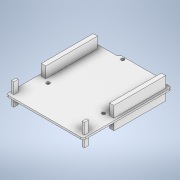
# Autodesk Inventor part: Microcontroller
Saved by Autodesk Inventor 2022 (Build 260153000, 153)
## iProperties
Created: 2022-02-18
Part Number: Microcontroller
Material: Generic
Document SubType Name: Modeling
Designer: woutr
Density: 1 g/cm^3
Appearance: White
Author: woutr
Autodesk Inventor part; units mm, degrees
ref_plane "YZ Plane" through (0, 0, 0) normal (1, 0, 0) x (0, 1, 0)
ref_plane "XZ Plane" through (0, 0, 0) normal (0, 1, 0) x (-1, 0, 0)
ref_plane "XY Plane" through (0, 0, 0) normal (0, 0, 1) x (1, 0, 0)
sketch "Sketch1" plane through (0, 0, 0) normal (0, 1, 0) x (-1, 0, 0)
  line L0 (0, 0) -> (70, 0)
  line L1 (70, 0) -> (70, -80.5)
  line L2 (70, -80.5) -> (49.49, -80.5)
  line L3 (0, 0) -> (0, -80.5)
  line L4 (0, -80.5) -> (11.33, -80.5)
  line L5 (47.54, -82.45) -> (13.28, -82.45)
  line L6 (49.49, -80.5) -> (47.54, -82.45)
  line L7 (11.33, -80.5) -> (13.28, -82.45)
  dimension "d0" = 70
  dimension "d1" = 80.5
  dimension "d2" = 20.51
  dimension "d3" = 80.5
  dimension "d4" = 11.33
  dimension "d5" = 82.45
  dimension "d6" = 45
  dimension "d7" = 45
  constraints: 16 end point, 3 perpendicular, 2 horizontal, 1 vertical
  measures "d0" distance of L0.start L0.end
  measures "d1" distance of L0.end L1.end
  measures "d2" distance of L1.end L2.end
  measures "d3" distance of L0.start L3.end
  measures "d4" distance of L3.end L4.end
  measures "d5" distance between parallel lines of L0 L5
  measures "d6" angle of L2 L6
  measures "d7" angle of L4 L7
extrude "Extrusion1" add sketch "Sketch1" along normal blind 1.65
fillet "Fillet1" radius 2 4 edges at (0, 0.825, 0) (-70, 0.825, 0) (0, 0.825, -80.5) (-70, 0.825, -80.5)
sketch "Sketch2" plane through (0, 1.65, 0) normal (0, 1, 0) x (1, 0, 0)
  circle A0 centre (-59.5, 27.7) radius 1.5
  circle A1 centre (-10.5, 29) radius 1.5
  circle A2 centre (-44.2, 80.15) radius 1.5
  line L0 (-68, 0) -> (-2, 0) projected
  line L1 (0, 2) -> (0, 78.5) projected
  line L2 (-70, 78.5) -> (-70, 2) projected
  line L3 (-13.28, 82.45) -> (-47.54, 82.45) projected
  point P0 (0, 0)
  dimension "d11" = 3
  dimension "d12" = 3
  dimension "d13" = 3
  dimension "d14" = 29
  dimension "d15" = 10.5
  dimension "d16" = 10.5
  dimension "d17" = 2.3
  dimension "d18" = 25.8
  dimension "d40" = 27.7
  constraints: 3 centre point
  measures "d11" diameter of A0
  measures "d12" diameter of A1
  measures "d13" diameter of A2
  measures "d14" distance from line of L0 A1.centre
  measures "d15" distance from line of L1 A1.centre
  measures "d16" distance from line of L2 A0.centre
  measures "d17" distance from line of L3 A2.centre
  measures "d18" distance from line of L2 A2.centre
  measures "d40" distance from line of L0 A0.centre
extrude "Extrusion2" cut sketch "Sketch2" against normal through all
sketch "Sketch3" plane through (0, 0, 0) normal (0, -1, 0) x (1, 0, 0)
  line L0 (-2, -30) -> (-6, -30)
  line L1 (-6, -30) -> (-6, -77)
  line L2 (-6, -77) -> (-2, -77)
  line L3 (-2, -77) -> (-2, -30)
  line L4 (-68, 0) -> (-2, 0) projected
  line L5 (0, -2) -> (0, -78.5) projected
  line L6 (-64, -30) -> (-68, -30)
  line L7 (-68, -30) -> (-68, -77)
  line L8 (-68, -77) -> (-64, -77)
  line L9 (-64, -77) -> (-64, -30)
  line L10 (-70, -78.5) -> (-70, -2) projected
  line L11 (-49.49, -80.5) -> (-68, -80.5) projected
  line L12 (-2, -7) -> (-4, -7)
  line L13 (-4, -7) -> (-4, -3)
  line L14 (-4, -3) -> (-2, -3)
  line L15 (-2, -3) -> (-2, -7)
  line L16 (-66, -7) -> (-68, -7)
  line L17 (-68, -7) -> (-68, -3)
  line L18 (-68, -3) -> (-66, -3)
  line L19 (-66, -3) -> (-66, -7)
  point P0 (0, 0)
  point P1 (-4, -77)
  point P2 (-66, -77)
  point P3 (-2, -5)
  point P4 (-68, -5)
  point P5 (-3, -3)
  point P6 (-67, -3)
  dimension "d21" = 4
  dimension "d22" = 47
  dimension "d23" = 30
  dimension "d24" = 2
  dimension "d27" = 2
  dimension "d28" = 4
  dimension "d30" = 30
  dimension "d33" = 2
  dimension "d34" = 4
  dimension "d35" = 2
  dimension "d36" = 4
  dimension "d37" = 3
  constraints: 32 end point, 8 parallel, 6 midpoint, 4 horizontal, 4 perpendicular, 2 horizontal alignment, 2 vertical alignment
  measures "d21" distance of L2.end L1.end
  measures "d22" distance of L1.end L0.end
  measures "d23" distance between parallel lines of L4 L0
  measures "d24" distance between parallel lines of L5 L3
  measures "d27" distance between parallel lines of L10 L7
  measures "d28" distance between parallel lines of L7 L9
  measures "d30" distance from line of L4 L6.start
  measures "d33" distance of L13.end L14.end
  measures "d34" distance of L12.end L13.end
  measures "d35" distance of L17.end L18.end
  measures "d36" distance of L16.end L17.end
  measures "d37" distance from line of L4 point (-3, -3)
extrude "Extrusion3" add sketch "Sketch3" along normal blind 8.3
sketch "Sketch4" plane through (0, 1.65, 0) normal (0, 1, 0) x (1, 0, 0)
  line L0 (-2, 77) -> (-2, 30) projected
  line L1 (-6, 30) -> (-6, 77) projected
  line L2 (-2, 77) -> (-6, 77)
  line L3 (-6, 77) -> (-6, 30)
  line L4 (-6, 30) -> (-2, 30)
  line L5 (-2, 30) -> (-2, 77)
  line L6 (-64, 77) -> (-64, 30) projected
  line L7 (-68, 77) -> (-68, 30) projected
  line L8 (-64, 77) -> (-68, 77)
  line L9 (-68, 77) -> (-68, 30)
  line L10 (-68, 30) -> (-64, 30)
  line L11 (-64, 30) -> (-64, 77)
  line L12 (-66, 3) -> (-66, 7) projected
  line L13 (-68, 3) -> (-68, 7) projected
  line L14 (-66, 3) -> (-68, 3)
  line L15 (-68, 3) -> (-68, 7)
  line L16 (-68, 7) -> (-66, 7)
  line L17 (-66, 7) -> (-66, 3)
  line L18 (-2, 3) -> (-2, 7) projected
  line L19 (-4, 7) -> (-4, 3) projected
  line L20 (-2, 3) -> (-4, 3)
  line L21 (-4, 3) -> (-4, 7)
  line L22 (-4, 7) -> (-2, 7)
  line L23 (-2, 7) -> (-2, 3)
  point P0 (0, 0)
  constraints: 32 end point, 8 parallel, 4 horizontal, 4 perpendicular
extrude "Extrusion4" add sketch "Sketch4" along normal blind 10
body "Solid1"
